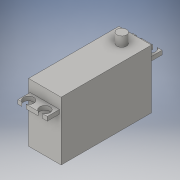
# Autodesk Inventor part: Serial Motor
Saved by Autodesk Inventor 2016 (Build 200138000, 138)
## iProperties
Created: 2016-10-05
Part Number: Serial Motor
Material: Generic
Document SubType Name: Modeling
Designer: sheehm
Density: 1 g/cm^3
Appearance: Default
Author: sheehm
Autodesk Inventor part; units mm, degrees
ref_plane "YZ Plane" through (0, 0, 0) normal (1, 0, 0) x (0, 1, 0)
ref_plane "XZ Plane" through (0, 0, 0) normal (0, 1, 0) x (-1, 0, 0)
ref_plane "XY Plane" through (0, 0, 0) normal (0, 0, 1) x (1, 0, 0)
sketch "Sketch5" plane through (0, 0, 0) normal (1, 0, 0) x (0, 1, 0)
  point P0 (0, 0)
sketch "Sketch6" plane through (0, 0, 0) normal (0, 1, 0) x (-1, 0, 0)
  line L0 (7.2949, 6.399) -> (-12.7051, 6.399)
  line L1 (-12.7051, 6.399) -> (-12.7051, -49.101)
  line L2 (-12.7051, -49.101) -> (7.2949, -49.101)
  line L3 (7.2949, -49.101) -> (7.2949, 6.399)
  point P0 (0, 0)
  dimension "d18" = 20
  dimension "d19" = 55.5
  constraints: 8 end point, 2 parallel, 1 horizontal, 1 perpendicular
  measures "d18" distance of L2.end L1.end
  measures "d19" distance of L1.end L0.end
extrude "Extrusion4" add sketch "Sketch6" along normal blind 36.1
sketch "Sketch7" plane through (-7.2949, 0, 6.399) normal (0, 0, 1) x (1, 0, 0)
  line L0 (0, 0) -> (0, 36.1) projected
  line L1 (20, 0) -> (20, 36.1) projected
  line L2 (1, 26.6) -> (19, 26.6)
  line L3 (19, 26.6) -> (19, 29.1)
  line L4 (19, 29.1) -> (1, 29.1)
  line L5 (1, 29.1) -> (1, 26.6)
  point P0 (7.2949, 0)
  dimension "d25" = 2.5
  constraints: 8 end point, 2 parallel, 1 horizontal, 1 perpendicular
  measures "d25" distance of L3.end L2.end
extrude "Extrusion5" add sketch "Sketch7" along normal blind 7.5
sketch "Sketch8" plane through (12.7051, 0, -49.101) normal (0, 0, -1) x (-1, 0, 0)
  line L0 (0, 0) -> (0, 36.1) projected
  line L1 (1, 26.6) -> (19, 26.6) projected
  line L2 (1, 26.6) -> (19, 26.6)
  line L3 (19, 26.6) -> (19, 29.1) projected
  line L4 (19, 26.6) -> (19, 29.1)
  line L5 (19, 29.1) -> (1, 29.1) projected
  line L6 (19, 29.1) -> (1, 29.1)
  line L7 (1, 29.1) -> (1, 26.6) projected
  line L8 (1, 29.1) -> (1, 26.6)
  point P0 (12.7051, 0)
  constraints: 8 end point, 4 collinear
extrude "Extrusion6" add sketch "Sketch8" along normal blind 7.5
sketch "Sketch9" plane through (0, 36.1, 0) normal (0, 1, 0) x (1, 0, 0)
  line L0 (12.7051, -6.399) -> (12.7051, 49.101) projected
  line L1 (-7.2949, 49.101) -> (-7.2949, -6.399) projected
  circle A0 centre (2.7051, 40.851) radius 2.95
  line L2 (12.7051, 49.101) -> (-7.2949, 49.101) projected
  point P0 (0, 0)
  dimension "d35" = 5.9
  dimension "d39" = 10
  dimension "d40" = 8.25
  constraints: 1 centre point
  measures "d35" diameter of A0
  measures "d39" distance from line of L0 A0.centre
  measures "d40" distance from line of L2 A0.centre
extrude "Extrusion7" add sketch "Sketch9" along normal blind 6
sketch "Sketch11" plane through (-6.2949, 29.1, 6.399) normal (0, 1, 0) x (1, 0, 0)
  line L0 (-1, 0) -> (19, 0) projected
  line L1 (10, -4) -> (10, 0)
  line L2 (8, -4) -> (8, 0)
  line L3 (10, -4) -> (8, -4)
  line L4 (18, 0) -> (18, -7.5) projected
  circle A0 centre (13.6676, -4.63) radius 2.25
  circle A1 centre (3.6676, -4.63) radius 2.25
  point P0 (6.2949, 6.399)
  point P1 (0, -7.5)
  dimension "d48" = 4.5
  dimension "d50" = 4.5
  constraints: 6 end point, 2 centre point, 2 point on line, 1 horizontal, 1 perpendicular, 1 vertical
  measures "d48" diameter of A0
  measures "d50" diameter of A1
hole "Hole1" at (-2.6273, 29.1, 11.029) at (7.3727, 29.1, 11.029) direction (0, -1, 0) diameter 6.35 end through all
sketch "Sketch15" plane through (-6.2949, 29.1, -49.101) normal (0, 1, 0) x (1, 0, 0)
  circle A0 centre (13.6566, 4.6228) radius 2.25
  circle A1 centre (3.6566, 4.6228) radius 2.25
  point P0 (6.2949, -49.101)
  point P1 (18, 0)
  dimension "d64" = 4.5
  dimension "d66" = 4.5
  constraints: 2 centre point
  measures "d64" diameter of A0
  measures "d66" diameter of A1
hole "Hole2" at (-2.6383, 29.1, -53.7238) at (7.3617, 29.1, -53.7238) direction (0, -1, 0) diameter 6.35 end through all
body "Solid2"
